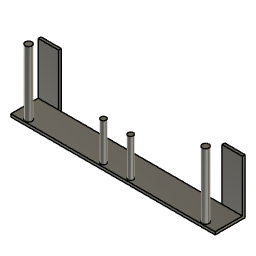
maintien_livre v2 (Autodesk Fusion 360 design; units mm, degrees)
Autodesk Fusion 360 part; units mm, degrees
sketch "Esquisse1" plane through (0, 0, 0) normal (0, 0, 1) x (1, 0, 0)
  line L0 (0, 0) -> (150, 0)
  line L1 (150, 0) -> (150, 20)
  line L2 (150, 20) -> (0, 20)
  line L3 (0, 20) -> (0, 0)
  line L4 (0, 20) -> (15, 20)
  line L5 (15, 20) -> (15, 22)
  line L6 (15, 22) -> (0, 22)
  line L7 (0, 22) -> (0, 20)
  line L8 (150, 20) -> (135, 20)
  line L9 (135, 20) -> (135, 22)
  line L10 (135, 22) -> (150, 22)
  line L11 (150, 22) -> (150, 20)
  line L12 (75, 0) -> (75, 20)
  circle A0 centre (10, 3) radius 2.5
  circle A1 centre (140, 3) radius 2.5
  circle A2 centre (85, 3) radius 2
  circle A3 centre (65, 3) radius 2
  dimension "d13" = 150
  dimension "d14" = 20
  dimension "d15" = 5
  dimension "d16" = 5
  dimension "d17" = 4
  dimension "d18" = 4
  dimension "d19" = 10
  dimension "d20" = 10
  dimension "d21" = 10
  dimension "d22" = 10
  dimension "d23" = 3
  dimension "d24" = 3
  dimension "d25" = 3
  dimension "d26" = 3
  dimension "d27" = 2
  dimension "d28" = 15
  dimension "d29" = 15
  dimension "d30" = 2
  constraint horizontal L0
  constraint vertical L1
  constraint horizontal L2
  constraint vertical L3
  constraint coincident L0.start L3.end
  constraint horizontal L4
  constraint vertical L5
  constraint horizontal L6
  constraint vertical L7
  constraint horizontal L8
  constraint vertical L9
  constraint horizontal L10
  constraint vertical L11
  constraint midpoint L0 L12.start
  constraint midpoint L2 L12.end
  measures "d13" distance of L0.start L0.end
  measures "d14" distance of L0.start L2.end
  measures "d15" diameter of A0
  measures "d16" diameter of A1
  measures "d17" diameter of A2
  measures "d18" diameter of A3
  measures "d19" distance of L3 A0.centre
  measures "d20" distance of L1 A1.centre
  measures "d21" distance of L12 A2.centre
  measures "d22" distance of L12 A3.centre
  measures "d23" distance of L0 A0.centre
  measures "d24" distance of L0 A3.centre
  measures "d25" distance of L0 A2.centre
  measures "d26" distance of L0 A1.centre
  measures "d27" distance of L4.end L5.end
  measures "d28" distance of L5.end L6.end
  measures "d29" distance of L9.end L10.end
  measures "d30" distance of L8.end L9.end
extrude "Extrusion1" add sketch "Esquisse1" along normal blind 40 contours L2 L4 L5 L6 L7 | L2 L8 L9 L10 L11 makes body 1 at (145, 20, 26.6667) makes body 2 at (10, 22, 26.6667)
extrude "Extrusion2" add sketch "Esquisse1" along normal blind 50 separate body contours A0 | A1 makes body 3 at (12.4876, 2.7511, 16.6667) makes body 4 at (140.6771, 5.4066, 33.3333)
extrude "Extrusion3" add sketch "Esquisse1" along normal blind 30 separate body contours A2 | A3 makes body 5 at (66.3234, 4.4996, 20) makes body 6 at (83.6035, 4.4317, 20)
extrude "Extrusion4" add sketch "Esquisse1" along normal blind 2 contours L0 L2 L3 L4 L12 | L0 L1 L2 L8 L12 bodies 1 2 3 4 5 6
equation "longueur_totale = 150 mm"
equation "largeur_totale = 20 mm"
equation "hauteur_base = 2 mm"
equation "hauteur_plaque_maintien = 40 mm"
equation "hauteur_tube_ext = 50 mm"
equation "hauteur_tube_int = 30 mm"
equation "rayon_tube_ext = 5 mm"
equation "rayon_tube_int = 4 mm"
equation "longueur_plaque_maintien = 15 mm"
equation "largeur_plaque_maintien = 2 mm"
equation "ecart_tube_ext_extérieur = 10 mm"
equation "ecart_tube_int_centre = 10 mm"
equation "d13 = longueur_totale"
equation "d14 = largeur_totale"
equation "d15 = rayon_tube_ext"
equation "d16 = rayon_tube_ext"
equation "d17 = rayon_tube_int"
equation "d18 = rayon_tube_int"
equation "d19 = ecart_tube_ext_extérieur"
equation "d20 = ecart_tube_ext_extérieur"
equation "d21 = ecart_tube_int_centre"
equation "d22 = ecart_tube_int_centre"
equation "d24 = d23"
equation "d25 = d23"
equation "d26 = d23"
equation "d27 = largeur_plaque_maintien"
equation "d28 = longueur_plaque_maintien"
equation "d29 = longueur_plaque_maintien"
equation "d30 = largeur_plaque_maintien"
equation "d31 = hauteur_plaque_maintien"
equation "d33 = hauteur_tube_ext"
equation "d35 = hauteur_tube_int"
equation "d37 = hauteur_base"
